mount to mold v1 (Autodesk Fusion 360 design; units mm, degrees)
Autodesk Fusion 360 part; units mm, degrees
sketch "Sketch1" plane through (0, 0, 0) normal (0, 1, 0) x (1, 0, 0)
  line L0 (50, -25) -> (-50, -25)
  line L1 (-50, -25) -> (-50, 25)
  line L2 (-50, 25) -> (50, 25)
  line L3 (50, 25) -> (50, -25)
  line L4 (50, -25) -> (-50, 25) construction
  line L5 (-50, -25) -> (50, 25) construction
  dimension "d1" = 100
  dimension "d2" = 50
  constraint horizontal L0
  constraint perpendicular L0 L1
  constraint parallel L0 L2
  constraint parallel L1 L3
  constraint coincident L4 origin
  constraint coincident L5 origin
  measures "d1" distance of L1.end L2.end
  measures "d2" distance of L0.end L1.end
extrude "Extrude1" add sketch "Sketch1" along normal blind 65
sketch "Sketch2" plane through (0, 0, 25) normal (0, 0, 1) x (1, 0, 0)
  line L0 (-50, 0) -> (50, 0)
  line L1 (50, 0) -> (50, 65)
  line L2 (50, 65) -> (-50, 65)
  line L3 (-50, 65) -> (-50, 0)
  line L4 (-50, 0) -> (50, 0)
  line L5 (50, 0) -> (50, 15)
  line L6 (50, 15) -> (-50, 15)
  line L7 (-50, 15) -> (-50, 0)
  line L8 (-40, 15) -> (-50, 15)
  line L9 (-50, 15) -> (-50, 65)
  line L10 (-50, 65) -> (-40, 65)
  line L11 (40, 15) -> (50, 15)
  line L12 (50, 15) -> (50, 65)
  line L13 (50, 65) -> (40, 65)
  line L14 (-10, 65) -> (10, 65)
  line L15 (10, 65) -> (10, 15)
  line L16 (10, 15) -> (-10, 15)
  line L17 (-10, 15) -> (-10, 65)
  line L18 (10, 65) -> (30, 65)
  line L19 (30, 65) -> (30, 15)
  line L20 (30, 15) -> (10, 15)
  line L21 (10, 15) -> (10, 65)
  line L22 (-10, 65) -> (-30, 65)
  line L23 (-30, 65) -> (-30, 15)
  line L24 (-30, 15) -> (-10, 15)
  line L25 (-10, 15) -> (-10, 65)
  line L26 (-30, 65) -> (-50, 65)
  line L27 (-50, 65) -> (-50, 15)
  line L28 (-50, 15) -> (-30, 15)
  line L29 (-30, 15) -> (-30, 65)
  line L30 (30, 65) -> (50, 65)
  line L31 (50, 65) -> (50, 15)
  line L32 (50, 15) -> (30, 15)
  line L33 (30, 15) -> (30, 65)
  dimension "d5" = 100
  dimension "d6" = 15
  dimension "d7" = 20
  dimension "d8" = 20
  dimension "d9" = 20
  dimension "d10" = 20
  dimension "d11" = 20
  constraint horizontal L4
  constraint vertical L5
  constraint horizontal L6
  constraint vertical L7
  constraint coincident L0.start L3.end
  constraint horizontal L8
  constraint vertical L9
  constraint horizontal L10
  constraint coincident L2.end L3.start
  constraint coincident L6 L8.start
  constraint horizontal L11
  constraint vertical L12
  constraint horizontal L13
  constraint coincident L1.end L2.start
  constraint coincident L6 L11.start
  constraint horizontal L14
  constraint vertical L15
  constraint horizontal L16
  constraint vertical L17
  constraint coincident L6 L15.end
  constraint coincident L2 L14.start
  constraint horizontal L18
  constraint vertical L19
  constraint horizontal L20
  constraint vertical L21
  constraint coincident L6 L19.end
  constraint horizontal L22
  constraint vertical L23
  constraint horizontal L24
  constraint vertical L25
  constraint coincident L6 L23.end
  constraint horizontal L26
  constraint vertical L27
  constraint horizontal L28
  constraint vertical L29
  constraint horizontal L30
  constraint vertical L31
  constraint horizontal L32
  constraint vertical L33
  measures "d5" distance of L0.start L0.end
  measures "d6" distance of L0.start L6.end
  measures "d7" distance of L17 L23
  measures "d8" distance of L15 L25
  measures "d9" distance of L15 L33
  measures "d10" distance of L12 L19
  measures "d11" distance of L22.end L2.end
extrude "Extrude2" cut sketch "Sketch2" against normal blind 50 contours L2 L6 L17 L22 L23 L24 L25 L29 | L2 L6 L15 L18 L19 L20 L21 L33
sketch "Sketch3" plane through (-50, 0, 0) normal (-1, 0, 0) x (0, 0, 1)
  line L0 (-25, 0) -> (25, 0)
  line L1 (25, 0) -> (25, 65)
  line L2 (25, 65) -> (-25, 65)
  line L3 (-25, 65) -> (-25, 0)
  circle A0 centre (0, 40) radius 25
  dimension "d14" = 50
  dimension "d15" = 40
  constraint tangent L3 A0
  measures "d14" diameter of A0
  measures "d15" distance of L0 A0.centre
extrude "Extrude3" cut sketch "Sketch3" against normal blind 100 contours L2 L3 A0 | L1 L2 A0
sketch "Sketch4" plane through (-50, 0, 0) normal (-1, 0, 0) x (0, 0, 1)
  arc A0 (25, 40) -> (-25, 40) centre (0, 40) ccw
  line L0 (-25, 40) -> (-25, 0)
  line L1 (-25, 0) -> (25, 0)
  line L2 (25, 0) -> (25, 40)
  line L3 (0, 40) -> (0, 0)
  constraint coincident A0.centre L3.start
  constraint coincident L3.end origin
hole "Hole1" at (-50, 40, 0) direction (1, 0, 0) diameter 25 end through all
sketch "Sketch5" plane through (0, 15, 0) normal (0, 1, 0) x (-1, 0, 0)
  line L0 (30, 25) -> (10, 25)
  line L1 (10, 25) -> (10, -25)
  line L2 (10, -25) -> (30, -25)
  line L3 (30, -25) -> (30, 25)
  line L4 (20, 0) -> (20, -25)
  line L5 (-20, 0) -> (-20, -25)
  dimension "d21" = 25
  dimension "d22" = 40
  constraint midpoint L2 L4.end
  constraint perpendicular L2 L4
  constraint perpendicular L2 L5
  measures "d21" distance of L5.start L5.end
  measures "d22" distance of L4 L5
hole "Hole2" at (-20, 15, 0) at (20, 15, 0) direction (0, -1, 0) diameter 10 depth 100 tip angle 118 counterbore diameter 16 counterbore depth 10
